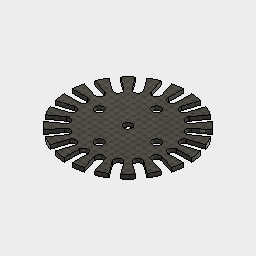
Wheel Front Plate (Autodesk Fusion 360 design; units mm, degrees)
Autodesk Fusion 360 part; units mm, degrees
note: some values were not read from the file. Set by a fixed rule: which sketch regions a step uses.
sketch "Sketch1" plane through (0, 0, 0) normal (0, 1, 0) x (1, 0, 0)
  line L0 (-1.6, -22.443) -> (-1.6, -22.9443)
  line L1 (1.6, -17.1) -> (1.6, -22.443)
  line L2 (12.8937, 11.3456) -> (17.2163, 14.4861)
  line L3 (15.7686, 6.8059) -> (20.8502, 8.457)
  line L4 (0, 15.5) -> (0, 15.5)
  arc A0 (-17.6219, -14.7807) -> (-14.7807, -17.6219) centre (0, 0) ccw
  arc A1 (-12.8937, -11.3456) -> (-12.5398, -9.1107) centre (-13.8342, -10.0511) ccw
  arc A2 (-12.5398, -9.1107) -> (-14.7746, -8.7567) centre (-13.8342, -10.0511) ccw
  arc A3 (-15.7686, -6.8059) -> (-14.7414, -4.7898) centre (-16.2631, -5.2842) ccw
  arc A4 (-14.7414, -4.7898) -> (-16.7575, -3.7625) centre (-16.2631, -5.2842) ccw
  circle A5 centre (11, 0) radius 1.6
  arc A6 (15.5, 0) -> (17.1, -1.6) centre (17.1, 0) ccw
  arc A7 (17.1, 1.6) -> (15.5, 0) centre (17.1, 0) ccw
  arc A8 (-8.6119, 21.3269) -> (-12.1919, 19.5028) centre (0, 0) ccw
  arc A9 (-14.7807, 17.6219) -> (-17.6219, 14.7807) centre (0, 0) ccw
  arc A10 (-19.5028, 12.1919) -> (-21.3269, 8.6119) centre (0, 0) ccw
  line L5 (-20.8502, 8.457) -> (-21.3269, 8.6119)
  line L6 (-17.2163, 14.4861) -> (-17.6219, 14.7807)
  line L7 (-1.6, -22.443) -> (-1.6, -17.1)
  line L8 (6.8059, -15.7686) -> (8.457, -20.8502)
  arc A11 (6.8059, -15.7686) -> (4.7898, -14.7414) centre (5.2842, -16.2631) ccw
  arc A12 (4.7898, -14.7414) -> (3.7625, -16.7575) centre (5.2842, -16.2631) ccw
  arc A13 (1.6, -17.1) -> (0, -15.5) centre (0, -17.1) ccw
  line L9 (17.1, 1.6) -> (22.443, 1.6)
  circle A14 centre (-11, 0) radius 1.6
  circle A15 centre (0, 0) radius 1.6
  arc A16 (-14.7414, 4.7898) -> (-15.7686, 6.8059) centre (-16.2631, 5.2842) ccw
  arc A17 (-16.7575, 3.7625) -> (-14.7414, 4.7898) centre (-16.2631, 5.2842) ccw
  arc A18 (-15.5, 0) -> (-17.1, 1.6) centre (-17.1, 0) ccw
  arc A19 (-17.1, -1.6) -> (-15.5, 0) centre (-17.1, 0) ccw
  arc A20 (-22.3157, 5.5685) -> (-22.9443, 1.6) centre (0, 0) ccw
  line L10 (-22.443, 1.6) -> (-22.9443, 1.6)
  line L11 (-22.443, -1.6) -> (-22.9443, -1.6)
  line L12 (-21.839, 5.4136) -> (-22.3157, 5.5685)
  line L13 (-22.443, 1.6) -> (-17.1, 1.6)
  line L14 (-17.1, -1.6) -> (-22.443, -1.6)
  line L15 (-16.7575, 3.7625) -> (-21.839, 5.4136)
  circle A21 centre (0, 11) radius 1.6
  arc A22 (12.5398, 9.1107) -> (14.7746, 8.7567) centre (13.8342, 10.0511) ccw
  arc A23 (12.8937, 11.3456) -> (12.5398, 9.1107) centre (13.8342, 10.0511) ccw
  arc A24 (9.1107, 12.5398) -> (11.3456, 12.8937) centre (10.0511, 13.8342) ccw
  arc A25 (8.7567, 14.7746) -> (9.1107, 12.5398) centre (10.0511, 13.8342) ccw
  arc A26 (4.7898, 14.7414) -> (6.8059, 15.7686) centre (5.2842, 16.2631) ccw
  arc A27 (3.7625, 16.7575) -> (4.7898, 14.7414) centre (5.2842, 16.2631) ccw
  arc A28 (17.6219, 14.7807) -> (14.7807, 17.6219) centre (0, 0) ccw
  arc A29 (12.1919, 19.5028) -> (8.6119, 21.3269) centre (0, 0) ccw
  arc A30 (5.5685, 22.3157) -> (1.6, 22.9443) centre (0, 0) ccw
  arc A31 (21.3269, 8.6119) -> (19.5028, 12.1919) centre (0, 0) ccw
  line L16 (1.6, 22.443) -> (1.6, 22.9443)
  line L17 (8.457, 20.8502) -> (8.6119, 21.3269)
  line L18 (5.4136, 21.839) -> (5.5685, 22.3157)
  line L19 (14.4861, 17.2163) -> (14.7807, 17.6219)
  line L20 (11.8973, 19.0973) -> (12.1919, 19.5028)
  arc A32 (-3.7625, -16.7575) -> (-4.7898, -14.7414) centre (-5.2842, -16.2631) ccw
  arc A33 (-22.9443, -1.6) -> (-22.3157, -5.5685) centre (0, 0) ccw
  line L21 (19.0973, 11.8973) -> (19.5028, 12.1919)
  line L22 (17.2163, 14.4861) -> (17.6219, 14.7807)
  line L23 (20.8502, 8.457) -> (21.3269, 8.6119)
  arc A34 (14.7414, 4.7898) -> (16.7575, 3.7625) centre (16.2631, 5.2842) ccw
  arc A35 (15.7686, 6.8059) -> (14.7414, 4.7898) centre (16.2631, 5.2842) ccw
  arc A36 (22.9443, 1.6) -> (22.3157, 5.5685) centre (0, 0) ccw
  line L24 (21.839, 5.4136) -> (22.3157, 5.5685)
  line L25 (22.443, -1.6) -> (22.9443, -1.6)
  line L26 (22.443, 1.6) -> (22.9443, 1.6)
  line L27 (21.839, 5.4136) -> (16.7575, 3.7625)
  line L28 (22.443, -1.6) -> (17.1, -1.6)
  line L29 (8.457, 20.8502) -> (6.8059, 15.7686)
  line L30 (3.7625, 16.7575) -> (5.4136, 21.839)
  line L31 (14.4861, 17.2163) -> (11.3456, 12.8937)
  line L32 (8.7567, 14.7746) -> (11.8973, 19.0973)
  line L33 (19.0973, 11.8973) -> (14.7746, 8.7567)
  line L34 (-19.0973, 11.8973) -> (-19.5028, 12.1919)
  line L35 (-11.8973, 19.0973) -> (-12.1919, 19.5028)
  line L36 (-14.4861, 17.2163) -> (-14.7807, 17.6219)
  line L37 (-5.4136, 21.839) -> (-5.5685, 22.3157)
  line L38 (-8.457, 20.8502) -> (-8.6119, 21.3269)
  line L39 (-1.6, 22.443) -> (-1.6, 22.9443)
  line L40 (-20.8502, 8.457) -> (-15.7686, 6.8059)
  line L41 (-17.2163, 14.4861) -> (-12.8937, 11.3456)
  line L42 (-14.7746, 8.7567) -> (-19.0973, 11.8973)
  line L43 (-11.8973, 19.0973) -> (-8.7567, 14.7746)
  line L44 (-11.3456, 12.8937) -> (-14.4861, 17.2163)
  line L45 (-5.4136, 21.839) -> (-3.7625, 16.7575)
  line L46 (-6.8059, 15.7686) -> (-8.457, 20.8502)
  line L47 (-1.6, 17.1) -> (-1.6, 22.443)
  line L48 (1.6, 22.443) -> (1.6, 17.1)
  arc A37 (-4.7898, 14.7414) -> (-3.7625, 16.7575) centre (-5.2842, 16.2631) ccw
  arc A38 (-6.8059, 15.7686) -> (-4.7898, 14.7414) centre (-5.2842, 16.2631) ccw
  arc A39 (-9.1107, 12.5398) -> (-8.7567, 14.7746) centre (-10.0511, 13.8342) ccw
  arc A40 (-11.3456, 12.8937) -> (-9.1107, 12.5398) centre (-10.0511, 13.8342) ccw
  arc A41 (-12.5398, 9.1107) -> (-12.8937, 11.3456) centre (-13.8342, 10.0511) ccw
  arc A42 (-14.7746, 8.7567) -> (-12.5398, 9.1107) centre (-13.8342, 10.0511) ccw
  arc A43 (-1.6, 22.9443) -> (-5.5685, 22.3157) centre (0, 0) ccw
  arc A44 (-21.3269, -8.6119) -> (-19.5028, -12.1919) centre (0, 0) ccw
  arc A45 (-4.7898, -14.7414) -> (-6.8059, -15.7686) centre (-5.2842, -16.2631) ccw
  arc A46 (-8.7567, -14.7746) -> (-9.1107, -12.5398) centre (-10.0511, -13.8342) ccw
  arc A47 (-9.1107, -12.5398) -> (-11.3456, -12.8937) centre (-10.0511, -13.8342) ccw
  line L49 (8.457, -20.8502) -> (8.6119, -21.3269)
  line L50 (5.4136, -21.839) -> (5.5685, -22.3157)
  line L51 (14.4861, -17.2163) -> (14.7807, -17.6219)
  line L52 (11.8973, -19.0973) -> (12.1919, -19.5028)
  line L53 (19.0973, -11.8973) -> (19.5028, -12.1919)
  line L54 (17.2163, -14.4861) -> (17.6219, -14.7807)
  line L55 (21.839, -5.4136) -> (22.3157, -5.5685)
  line L56 (20.8502, -8.457) -> (21.3269, -8.6119)
  arc A48 (22.3157, -5.5685) -> (22.9443, -1.6) centre (0, 0) ccw
  arc A49 (19.5028, -12.1919) -> (21.3269, -8.6119) centre (0, 0) ccw
  arc A50 (14.7807, -17.6219) -> (17.6219, -14.7807) centre (0, 0) ccw
  arc A51 (8.6119, -21.3269) -> (12.1919, -19.5028) centre (0, 0) ccw
  arc A52 (1.6, -22.9443) -> (5.5685, -22.3157) centre (0, 0) ccw
  arc A53 (16.7575, -3.7625) -> (14.7414, -4.7898) centre (16.2631, -5.2842) ccw
  arc A54 (14.7414, -4.7898) -> (15.7686, -6.8059) centre (16.2631, -5.2842) ccw
  arc A55 (14.7746, -8.7567) -> (12.5398, -9.1107) centre (13.8342, -10.0511) ccw
  arc A56 (12.5398, -9.1107) -> (12.8937, -11.3456) centre (13.8342, -10.0511) ccw
  arc A57 (11.3456, -12.8937) -> (9.1107, -12.5398) centre (10.0511, -13.8342) ccw
  arc A58 (9.1107, -12.5398) -> (8.7567, -14.7746) centre (10.0511, -13.8342) ccw
  line L57 (5.4136, -21.839) -> (3.7625, -16.7575)
  line L58 (11.3456, -12.8937) -> (14.4861, -17.2163)
  line L59 (11.8973, -19.0973) -> (8.7567, -14.7746)
  line L60 (14.7746, -8.7567) -> (19.0973, -11.8973)
  line L61 (17.2163, -14.4861) -> (12.8937, -11.3456)
  line L62 (16.7575, -3.7625) -> (21.839, -5.4136)
  line L63 (20.8502, -8.457) -> (15.7686, -6.8059)
  line L64 (1.6, -22.443) -> (1.6, -22.9443)
  arc A59 (0, -15.5) -> (-1.6, -17.1) centre (0, -17.1) ccw
  circle A60 centre (0, -11) radius 1.6
  line L65 (-15.7686, -6.8059) -> (-20.8502, -8.457)
  line L66 (-21.839, -5.4136) -> (-16.7575, -3.7625)
  line L67 (-12.8937, -11.3456) -> (-17.2163, -14.4861)
  line L68 (-19.0973, -11.8973) -> (-14.7746, -8.7567)
  line L69 (-8.7567, -14.7746) -> (-11.8973, -19.0973)
  line L70 (-14.4861, -17.2163) -> (-11.3456, -12.8937)
  line L71 (-3.7625, -16.7575) -> (-5.4136, -21.839)
  line L72 (-8.457, -20.8502) -> (-6.8059, -15.7686)
  line L73 (-20.8502, -8.457) -> (-21.3269, -8.6119)
  line L74 (-21.839, -5.4136) -> (-22.3157, -5.5685)
  line L75 (-17.2163, -14.4861) -> (-17.6219, -14.7807)
  line L76 (-19.0973, -11.8973) -> (-19.5028, -12.1919)
  line L77 (-11.8973, -19.0973) -> (-12.1919, -19.5028)
  line L78 (-14.4861, -17.2163) -> (-14.7807, -17.6219)
  line L79 (-5.4136, -21.839) -> (-5.5685, -22.3157)
  line L80 (-8.457, -20.8502) -> (-8.6119, -21.3269)
  arc A61 (-5.5685, -22.3157) -> (-1.6, -22.9443) centre (0, 0) ccw
  arc A62 (-12.1919, -19.5028) -> (-8.6119, -21.3269) centre (0, 0) ccw
  arc A63 (-1.6, 17.1) -> (1.6, 17.1) centre (0, 17.1) ccw
  point P0 (1.6, 15.5)
  point P1 (-1.6, 15.5)
extrude "Extrude1" add sketch "Sketch1" along normal blind 1.5
